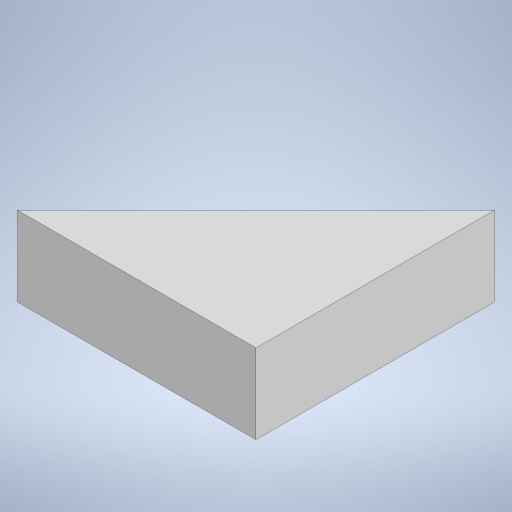
# Autodesk Inventor part: Treliça3
Saved by Autodesk Inventor 2023 (Build 270158000, 158)
## iProperties
Created: 2023-04-06
Part Number: Treliça3
Material: Generic
Document SubType Name: Sheet Metal
Designer: 062190003
Density: 1 g/cm^3
Sheet Metal Rule: Default_mm
Appearance: Default
Author: 062190003
Autodesk Inventor part; units mm, degrees
ref_plane "YZ Plane" through (0, 0, 0) normal (1, 0, 0) x (0, 1, 0)
ref_plane "XZ Plane" through (0, 0, 0) normal (0, 1, 0) x (-1, 0, 0)
ref_plane "XY Plane" through (0, 0, 0) normal (0, 0, 1) x (1, 0, 0)
sketch "Sketch1" plane through (0, 0, 0) normal (0, 1, 0) x (-1, 0, 0)
  line L0 (0, -15) -> (0, 0)
  line L1 (0, 0) -> (15, 0)
  line L2 (15, 0) -> (0, -15)
  dimension "d0" = 15
  constraints: 6 end point, 2 perpendicular, 1 vertical
  measures "d0" distance of L0.start L0.end
extrude "Extrusion1" add sketch "Sketch1" along normal blind 5
equation "\"BendRadius\" = Thickness"
equation "\"BendReliefWidth\" = Thickness"
equation "\"BendReliefDepth\" = 0.5 * Thickness"
equation "\"CornerReliefSize\" = 4 * Thickness"
equation "\"MinimumRemnant\" = 2 * Thickness"
equation "\"TransitionRadius\" = BendRadius"
equation "\"JacobiRadiusSize\" = BendRadius"
equation "\"GapSize\" = Thickness"
equation "\"Thickness\" = 0.5"
body "Solid1"
